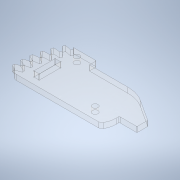
# Autodesk Inventor part: Laser-Pivot-Side
Saved by Autodesk Inventor 2021 (Build 250183000, 183)
## iProperties
Created: 2020-07-07
Part Number: Laser-Pivot-Side
Material: Acrylic, Clear
Document SubType Name: Modeling
Designer: lucas
Density: 1.19 g/cm^3
Appearance: Transparent - Clear
Project: 4Wire-Laser
Author: lucas
Revision Number: RLS_001
Autodesk Inventor part; units mm, degrees
ref_plane "YZ Plane" through (0, 0, 0) normal (1, 0, 0) x (0, 1, 0)
ref_plane "XZ Plane" through (0, 0, 0) normal (0, 1, 0) x (-1, 0, 0)
ref_plane "XY Plane" through (0, 0, 0) normal (0, 0, 1) x (1, 0, 0)
sketch "Sketch1" plane through (0, 0, 0) normal (0, 1, 0) x (-1, 0, 0)
  arc A0 (8.5698, -20.069) -> (12.1197, -20.3293) centre (11.6895, -1.861) ccw
  arc A1 (12.1197, -20.3293) -> (12.5731, -19.197) centre (-28.0196, -3.6) ccw
  arc A2 (12.5731, -19.197) -> (9.8246, -16.9353) centre (-0.4845, -32.2646) ccw
  arc A3 (9.8246, -16.9353) -> (10.1837, -15.8687) centre (-28.0196, -3.6) ccw
  arc A4 (10.1837, -15.8687) -> (13.7404, -15.7299) centre (11.2452, 2.5741) ccw
  arc A5 (13.7404, -15.7299) -> (14.0641, -14.554) centre (-28.0196, -3.6) ccw
  arc A6 (14.0641, -14.554) -> (11.0797, -12.6143) centre (2.5518, -29.0014) ccw
  arc A7 (11.0797, -12.6143) -> (11.3172, -11.5142) centre (-28.0196, -3.6) ccw
  arc A8 (11.3172, -11.5142) -> (14.8359, -10.978) centre (10.307, 6.9315) ccw
  arc A9 (14.8359, -10.978) -> (15.026, -9.7732) centre (-28.0196, -3.6) ccw
  arc A10 (15.026, -9.7732) -> (11.8431, -8.1799) centre (5.2036, -25.4188) ccw
  arc A11 (11.8431, -8.1799) -> (11.9559, -7.0601) centre (-28.0196, -3.6) ccw
  arc A12 (11.9559, -7.0601) -> (15.3925, -6.1333) centre (8.8868, 11.1565) ccw
  arc A13 (15.3925, -6.1333) -> (15.4465, -4.9148) centre (-28.0196, -3.6) ccw
  arc A14 (15.4465, -4.9148) -> (12.1053, -3.6879) centre (7.4376, -21.5618) ccw
  arc A15 (12.1053, -3.6879) -> (12.092, -2.5625) centre (-28.0196, -3.6) ccw
  arc A16 (12.092, -2.5625) -> (15.4032, -1.2568) centre (7.0026, 15.1959) ccw
  line L0 (-49.9112, -5.856) -> (-49.9112, -11.1707)
  line L1 (-49.6835, -11.59) -> (-38.0954, -19.1154)
  arc A17 (-38.0954, -19.1154) -> (-28.0196, -22.1) centre (-28.0196, -3.6) ccw
  line L2 (-28.0196, -22.1) -> (-6.4967, -22.1)
  arc A18 (-38.4504, 2.1104) -> (-39.9112, -3.6) centre (-28.0196, -3.6) ccw
  line L3 (-39.9112, -3.6) -> (-39.9112, -4.856)
  line L4 (-40.4112, -5.356) -> (-49.4112, -5.356)
  circle A19 centre (-28.0196, -3.6) radius 1.6
  arc A20 (6.7216, -26.0837) -> (5.8614, -25.0964) centre (-7.628, -37.7178) ccw
  arc A21 (5.8614, -25.0964) -> (6.4509, -24.1377) centre (-28.0196, -3.6) ccw
  arc A22 (6.4509, -24.1377) -> (9.9479, -24.8015) centre (11.6285, -6.4048) ccw
  arc A23 (9.9479, -24.8015) -> (10.5275, -23.7283) centre (-28.0196, -3.6) ccw
  arc A24 (10.5275, -23.7283) -> (8.0552, -21.1677) centre (-3.9362, -35.2201) ccw
  arc A25 (8.0552, -21.1677) -> (8.5698, -20.069) centre (-28.0196, -3.6) ccw
  arc A26 (-49.4112, -5.356) -> (-49.9112, -5.856) centre (-49.4112, -5.856) ccw
  arc A27 (-40.4112, -5.356) -> (-39.9112, -4.856) centre (-40.4112, -4.856) ccw
  line L5 (-6.2467, -22.35) -> (-6.2467, -25.6)
  arc A28 (15.4032, -1.2568) -> (15.3198, -0.0322) centre (-28.0196, -3.6) ccw
  arc A29 (15.3198, -0.0322) -> (13.9798, 0.3742) centre (9.2916, -17.4943) ccw
  arc A30 (-49.9112, -11.1707) -> (-49.6835, -11.59) centre (-49.4112, -11.1707) ccw
  line L6 (3.4804, -15.5) -> (6.4804, -15.5) construction
  line L7 (-6.2467, -25.6) -> (-6.2467, -23.3)
  line L8 (-28.0196, 0.5) -> (-39.182, 0.5) construction
  line L9 (-5.7467, -26.1) -> (6.7138, -26.1)
  arc A31 (6.7138, -26.1) -> (6.7216, -26.0837) centre (6.7138, -26.09) ccw
  line L10 (-28.0196, -3.6) -> (9.082, -27.6941) construction
  line L11 (-28.0196, -3.6) -> (16.219, -3.6) construction
  arc A32 (3.3753, -26.1) -> (10.6054, -3.6) centre (-28.0196, -3.6) ccw construction
  line L12 (-28.0196, -3.6) -> (1.3338, -22.6624) construction
  circle A33 centre (1.3338, -22.6624) radius 1.6
  line L13 (-28.0196, -3.6) -> (-28.0196, 3.15)
  line L14 (-36.6961, 3.15) -> (9.9746, 3.15)
  line L15 (6.4804, -3.5) -> (6.4804, -15.5) construction
  line L16 (3.4804, -3.5) -> (3.4804, -15.5) construction
  arc A34 (-36.6961, 3.15) -> (-38.4504, 2.1104) centre (-36.6961, 1.15) ccw
  line L17 (13.0794, 0.8884) -> (11.3826, 2.5704)
  arc A35 (11.3826, 2.5704) -> (9.9746, 3.15) centre (9.9746, 1.15) ccw
  arc A36 (13.0794, 0.8884) -> (13.9798, 0.3742) centre (14.4874, 2.3087) ccw
  arc A37 (-6.2467, -25.6) -> (-5.7467, -26.1) centre (-5.7467, -25.6) ccw
  arc A38 (-6.2467, -22.35) -> (-6.4967, -22.1) centre (-6.4967, -22.35) ccw
  line L18 (6.4804, -3.5) -> (3.4804, -3.5) construction
  line L19 (6.4904, -15.51) -> (3.4704, -15.51)
  line L20 (3.4704, -15.51) -> (3.4704, -3.49)
  line L21 (3.4704, -3.49) -> (6.4904, -3.49)
  line L22 (6.4904, -3.49) -> (6.4904, -15.51)
  arc A39 (3.7204, -3.49) -> (3.4704, -3.74) centre (3.4704, -3.49) ccw
  arc A40 (6.4904, -3.74) -> (6.2404, -3.49) centre (6.4904, -3.49) ccw
  arc A41 (3.4704, -15.26) -> (3.7204, -15.51) centre (3.4704, -15.51) ccw
  arc A42 (6.2404, -15.51) -> (6.4904, -15.26) centre (6.4904, -15.51) ccw
  line L23 (-18.9344, -9.5) -> (6.4804, -9.5) construction
  line L24 (-28.0196, -3.6) -> (-31.0196, -3.6) construction
  point P0 (-6.2467, -22.1)
  point P1 (-6.2467, -26.1)
  point P2 (6.7348, -26.1)
  point P3 (13.4712, 0.5)
  point P4 (-37.8098, 3.15)
  dimension "d0" = 0.5
  dimension "d2" = 0.5
  dimension "d17" = 33
  dimension "d18" = 33
  dimension "d19" = 38.625
  dimension "d20" = 35
  dimension "d21" = 3.2
  dimension "d22" = 6.75
  dimension "d24" = 2
  dimension "d25" = 2
  dimension "d26" = 0.5
  dimension "d27" = 0.25
  dimension "d28" = 34.5
  dimension "d30" = 0.01
  dimension "d31" = 0.25
  dimension "d32" = 0.25
  dimension "d33" = 0.25
  dimension "d34" = 0.25
  dimension "d39" = 6.75
  dimension "d40" = 6.65
  dimension "d41" = 12.65
  dimension "d43" = 12
  dimension "d44" = 3
  dimension "d45" = 21.7729
  dimension "d46" = 29.3535
  dimension "d56" = 25.2
  dimension "d57" = 25.25
  constraints: 85 point on circle, 50 end point, 43 centre point, 28 tangent, 20 point on line, 10 equal radius, 8 coincident, 6 horizontal, 3 parallel, 3 perpendicular, 2 vertical, 1 equal length, 1 midpoint, 55 other
  measures "d0" radius of A26
  measures "d2" radius of A30
  measures "d17" angle of L1 L2
  measures "d18" angle of L10 L11
  measures "d19" radius of A32
  measures "d20" distance of L10.start L12.end
  measures "d21" diameter of A33
  measures "d22" distance of L10.start L13.end
  measures "d24" radius of A34
  measures "d25" radius of A35
  measures "d26" radius of A37
  measures "d27" radius of A38
  measures "d28" distance from line of L10.start L15
  measures "d30" distance between parallel lines of L15 L22
  measures "d31" radius of A39
  measures "d32" radius of A40
  measures "d33" radius of A41
  measures "d34" radius of A42
  measures "d39" distance from line of A19.centre L14
  measures "d40" distance between parallel lines of L18 L14
  measures "d41" distance between parallel lines of L23 L14
  measures "d43" diameter of L18 L23
  measures "d44" distance of L15.start L16.start
  measures "d45" distance from line of L5 A32.centre
  measures "d46" horizontal distance of L12.end A32.centre
  measures "d56" diameter of L2 L23
  measures "d57" distance between parallel lines of L14 L2
extrude "Extrusion1" add sketch "Sketch1" along normal blind 3
body "Solid1"
